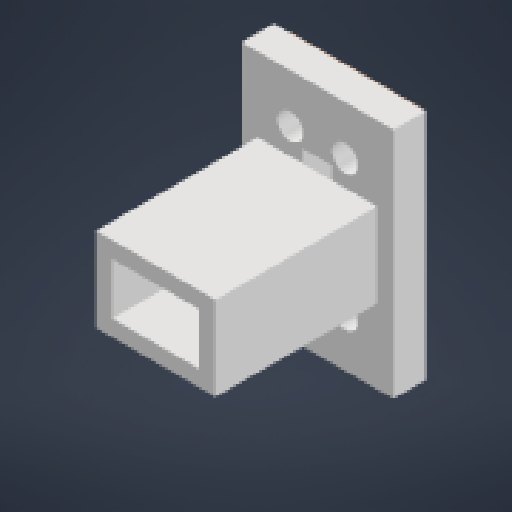
# Autodesk Inventor part: Tower
Saved by Autodesk Inventor 2024 (Build 280153000, 153)
## iProperties
Created: 2024-03-13
Part Number: Tower
Material: Generic
Document SubType Name: Modeling
Designer: Daniel
Density: 1 g/cm^3
Appearance: Default
Author: Daniel
Autodesk Inventor part; units mm, degrees
ref_plane "YZ Plane" through (0, 0, 0) normal (1, 0, 0) x (0, 1, 0)
ref_plane "XZ Plane" through (0, 0, 0) normal (0, 1, 0) x (-1, 0, 0)
ref_plane "XY Plane" through (0, 0, 0) normal (0, 0, 1) x (1, 0, 0)
ref_plane "Work Plane1" through (0, 0, 0) normal (0, 0, 1) x (1, 0, 0)
sketch "Sketch1" plane through (0, 0, 0) normal (0, 0, 1) x (1, 0, 0)
  line L0 (18.5, -31) -> (-18.5, -31) projected
  line L1 (18.5, 31) -> (18.5, -31) projected
  line L2 (-18.5, 31) -> (18.5, 31) projected
  line L3 (-18.5, -31) -> (-18.5, 31) projected
  circle A0 centre (8.5, -21) radius 3 projected
  line L4 (-4.5, 17) -> (-4.5, -17) projected
  line L5 (4.5, 17) -> (-4.5, 17) projected
  line L6 (4.5, -17) -> (4.5, 17) projected
  line L7 (-4.5, -17) -> (4.5, -17) projected
  circle A1 centre (-8.5, -21) radius 3 projected
  circle A2 centre (-8.5, 21) radius 3 projected
  circle A3 centre (8.5, 21) radius 3 projected
  circle A4 centre (-8.5, 21) radius 2.1
  line L8 (-8.5, 21) -> (-8.5, -21) construction
  line L9 (-8.5, -21) -> (-8.5, 21) construction
  line L10 (8.5, 21) -> (-8.5, 21) construction
  circle A5 centre (-8.5, -21) radius 2.1
  circle A6 centre (8.5, -21) radius 2.1
  circle A7 centre (8.5, 21) radius 2.1
  point P0 (0, 0)
  dimension "d8" = 4.2
  dimension "d9" = 42
  dimension "d10" = 17
  dimension "d11" = 4.2
  dimension "d12" = 4.2
  dimension "d13" = 4.2
  constraints: 6 end point, 4 centre point, 4 coincident, 1 collinear, 1 perpendicular, 1 vertical
  measures "d8" diameter of A4
  measures "d9" distance of L8.start L8.end
  measures "d10" distance of L10.start L8.start
  measures "d11" diameter of A5
  measures "d12" diameter of A6
  measures "d13" diameter of A7
ref_plane "Work Plane2" through (-77.3187, -62.8984, 2) normal (0, 0, 1) x (1, 0, 0)
extrude "Extrusion1" add sketch "Sketch1" along normal up to surface (2 mm away) contours L0 L3 L2 L1 | A0 | A1 | A2 | A3
sketch "Sketch2" plane through (-18.5, 31, 2) normal (0, 0, 1) x (1, 0, 0)
  line L0 (14, -14) -> (14, -48) projected
  line L1 (23, -14) -> (14, -14) projected
  line L2 (23, -48) -> (23, -14) projected
  line L3 (14, -48) -> (23, -48) projected
  line L4 (37, 0) -> (37, -62) projected
  line L5 (0, 0) -> (37, 0) projected
  line L6 (0, -62) -> (0, 0) projected
  line L7 (37, -62) -> (0, -62) projected
  line L8 (42, -67) -> (42, 5)
  line L9 (42, 5) -> (-5, 5)
  line L10 (-5, 5) -> (-5, -67)
  line L11 (-5, -67) -> (42, -67)
  circle A0 centre (10, -52) radius 2.1 projected
  circle A1 centre (27, -52) radius 2.1 projected
  circle A2 centre (10, -10) radius 2.1 projected
  circle A3 centre (27, -10) radius 2.1 projected
  line L12 (14, -14) -> (14, -48) projected
  line L13 (23, -14) -> (14, -14) projected
  line L14 (23, -48) -> (23, -14) projected
  line L15 (14, -48) -> (23, -48) projected
  line L16 (37, 0) -> (37, -62) projected
  line L17 (0, 0) -> (37, 0) projected
  line L18 (0, -62) -> (0, 0) projected
  line L19 (37, -62) -> (0, -62) projected
  circle A4 centre (27, -10) radius 4
  circle A5 centre (10, -10) radius 4
  circle A6 centre (27, -52) radius 4
  circle A7 centre (10, -52) radius 4
  point P0 (18.5, -31)
  dimension "d2" = 5
  dimension "d14" = 8
  dimension "d15" = 8
  dimension "d16" = 8
  dimension "d17" = 8
  constraints: 8 end point, 4 centre point, 4 coincident, 3 other
  measures "d2" distance between parallel lines of L4 L8
  measures "d14" diameter of A4
  measures "d15" diameter of A5
  measures "d16" diameter of A6
  measures "d17" diameter of A7
chamfer "Chamfer1" distance 1 angle 45 8 edges at (-18.5, 0, 0) (0, 31, 0) (-18.5, 31, 1) (18.5, 31, 1) (18.5, 0, 0) (18.5, -31, 1) (0, -31, 0) (-18.5, -31, 1)
extrude "Extrusion3" add sketch "Sketch2" along normal blind 10 contours L4 L7 L6 L5 | L11 L10 L9 L8
sketch "Sketch3" plane through (-18.5, 31, 12) normal (0, 0, 1) x (1, 0, 0)
  line L0 (37, -18) -> (0, -18)
  line L1 (0, -18) -> (0, -44)
  line L2 (0, -44) -> (37, -44)
  line L3 (37, -44) -> (37, -18)
  line L4 (42, -67) -> (42, 5) projected
  line L5 (-5, 5) -> (-5, -67) projected
  circle A0 centre (10, -52) radius 2.1 projected
  circle A1 centre (10, -10) radius 2.1 projected
  line L6 (32, -23) -> (5, -23)
  line L7 (5, -23) -> (5, -39)
  line L8 (5, -39) -> (32, -39)
  line L9 (32, -39) -> (32, -23)
  point P0 (18.5, -31)
  dimension "d20" = 5
  dimension "d21" = 5
  dimension "d22" = 8
  dimension "d23" = 8
  dimension "d24" = 5
  constraints: 16 end point, 4 parallel, 2 perpendicular, 1 horizontal, 3 other
  measures "d20" distance between parallel lines of L4 L3
  measures "d21" distance between parallel lines of L5 L1
  measures "d22" distance from line of A0.centre L2
  measures "d23" distance from line of A1.centre L0
  measures "d24" distance between parallel lines of L3 L9
extrude "Extrusion4" add sketch "Sketch3" along normal blind 50 contours L3 L2 L1 L0
chamfer "Chamfer2" distance 8 angle 45 4 edges at (-23.5, 0, 12) (0, -36, 12) (23.5, 0, 12) (0, 36, 12)
body "Solid1"
